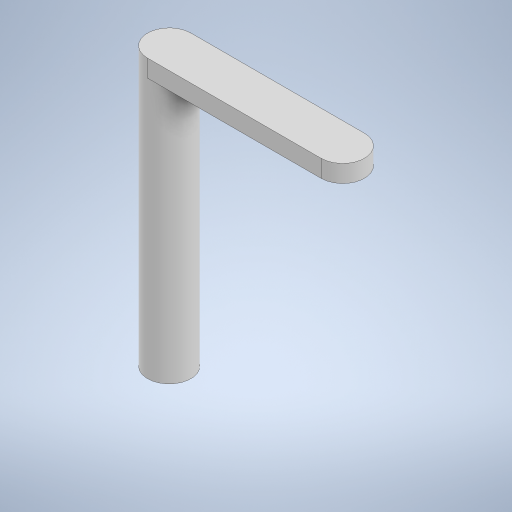
# Autodesk Inventor part: Motor_Arm
Saved by Autodesk Inventor 2024 (Build 280153000, 153)
## iProperties
Created: 2023-10-07
Part Number: Motor_Arm
Material: Generic
Document SubType Name: Modeling
Designer: tangl
Density: 1 g/cm^3
Appearance: Default
Author: tangl
Autodesk Inventor part; units mm, degrees
ref_plane "YZ Plane" through (0, 0, 0) normal (1, 0, 0) x (0, 1, 0)
ref_plane "XZ Plane" through (0, 0, 0) normal (0, 1, 0) x (-1, 0, 0)
ref_plane "XY Plane" through (0, 0, 0) normal (0, 0, 1) x (1, 0, 0)
sketch "Sketch1" plane through (0, 0, 0) normal (0, 1, 0) x (-1, 0, 0)
  circle A0 centre (0, 0) radius 6.35
  dimension "d0" = 12.7
  constraints: 1 centre point, 1 coincident
  measures "d0" diameter of A0
extrude "Extrusion1" add sketch "Sketch1" along normal blind 76.2
sketch "Sketch2" plane through (0, 76.2, 0) normal (0, 1, 0) x (1, 0, 0)
  arc A0 (0, 6.35) -> (0, -6.35) centre (0, 0) ccw
  line L0 (44.45, 0) -> (50.8, 0)
  arc A1 (50.8, -6.35) -> (50.8, 6.35) centre (50.8, 0) ccw
  line L1 (50.8, -6.35) -> (0, -6.35)
  line L2 (0, 6.35) -> (50.8, 6.35)
  dimension "d4" = 6.35
  dimension "d10" = 50.8
  dimension "d11" = 6.35
  dimension "d12" = 50.8
  dimension "d13" = 6.35
  constraints: 6 end point, 4 point on circle, 2 centre point, 2 coincident, 2 horizontal, 2 tangent, 1 parallel
  measures "d4" radius of A0
  measures "d10" distance of L0.end point (0, 0)
  measures "d11" radius of A1
  measures "d12" distance of L2.start L2.end
  measures "d13" distance from line of point (0, 0) L2
extrude "Extrusion2" add sketch "Sketch2" along normal blind 5.08
body "Solid1"
